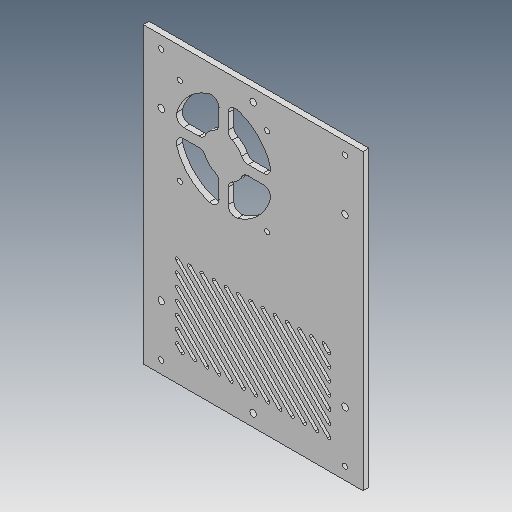
# Autodesk Inventor part: BREEZE-M05
Saved by Autodesk Inventor 2020 (Build 240168000, 168)
## iProperties
Created: 2020-04-12
Part Number: BREEZE-M05
Material: Generic
Description: BOTTOM PANEL
Document SubType Name: Modeling
Designer: John K
Density: 1 g/cm^3
Appearance: Default
Author: John K
Autodesk Inventor part; units mm, degrees
ref_plane "YZ Plane" through (0, 0, 0) normal (1, 0, 0) x (0, 1, 0)
ref_plane "XZ Plane" through (0, 0, 0) normal (0, 1, 0) x (-1, 0, 0)
ref_plane "XY Plane" through (0, 0, 0) normal (0, 0, 1) x (1, 0, 0)
sketch "Face" plane through (0, 0, 0) normal (0, 0, 1) x (1, 0, 0)
  arc A0 (60.9029, -217.5171) -> (63.1656, -215.2543) centre (62.0343, -216.3857) ccw
  arc A1 (29.1656, -161.2543) -> (26.9029, -163.5171) centre (28.0343, -162.3857) ccw
  arc A2 (29.1656, -181.2543) -> (26.9029, -183.5171) centre (28.0343, -182.3857) ccw
  line L0 (29.1656, -191.2543) -> (53.1656, -215.2543)
  arc A3 (50.9029, -217.5171) -> (53.1656, -215.2543) centre (52.0343, -216.3857) ccw
  line L1 (50.9029, -217.5171) -> (26.9029, -193.5171)
  arc A4 (29.1656, -191.2543) -> (26.9029, -193.5171) centre (28.0343, -192.3857) ccw
  line L2 (29.1656, -151.2543) -> (93.1656, -215.2543)
  line L3 (90.9029, -217.5171) -> (26.9029, -153.5171)
  line L4 (60.9029, -217.5171) -> (26.9029, -183.5171)
  line L5 (29.1656, -181.2543) -> (63.1656, -215.2543)
  line L6 (70.9029, -217.5171) -> (26.9029, -173.5171)
  arc A5 (29.1656, -201.2543) -> (26.9029, -203.5171) centre (28.0343, -202.3857) ccw
  line L7 (29.1656, -201.2543) -> (43.1656, -215.2543)
  line L8 (29.1656, -211.2543) -> (33.1656, -215.2543)
  line L9 (30.9029, -217.5171) -> (26.9029, -213.5171)
  line L10 (40.9029, -217.5171) -> (26.9029, -203.5171)
  arc A6 (90.9029, -217.5171) -> (93.1656, -215.2543) centre (92.0343, -216.3857) ccw
  arc A7 (150.9029, -157.5171) -> (153.1656, -155.2543) centre (152.0343, -156.3857) ccw
  line L11 (150.9029, -187.5171) -> (116.9029, -153.5171)
  line L12 (150.9029, -197.5171) -> (106.9029, -153.5171)
  line L13 (109.1656, -151.2543) -> (153.1656, -195.2543)
  line L14 (150.9029, -207.5171) -> (96.9029, -153.5171)
  line L15 (99.1656, -151.2543) -> (153.1656, -205.2543)
  line L16 (89.1656, -151.2543) -> (153.1656, -215.2543)
  line L17 (79.1656, -151.2543) -> (143.1656, -215.2543)
  line L18 (140.9029, -217.5171) -> (76.9029, -153.5171)
  line L19 (130.9029, -217.5171) -> (66.9029, -153.5171)
  line L20 (69.1656, -151.2543) -> (133.1656, -215.2543)
  arc A8 (120.9029, -217.5171) -> (123.1656, -215.2543) centre (122.0343, -216.3857) ccw
  arc A9 (130.9029, -217.5171) -> (133.1656, -215.2543) centre (132.0343, -216.3857) ccw
  arc A10 (140.9029, -217.5171) -> (143.1656, -215.2543) centre (142.0343, -216.3857) ccw
  arc A11 (150.9029, -217.5171) -> (153.1656, -215.2543) centre (152.0343, -216.3857) ccw
  arc A12 (110.9029, -217.5171) -> (113.1656, -215.2543) centre (112.0343, -216.3857) ccw
  arc A13 (150.9029, -187.5171) -> (153.1656, -185.2543) centre (152.0343, -186.3857) ccw
  arc A14 (150.9029, -197.5171) -> (153.1656, -195.2543) centre (152.0343, -196.3857) ccw
  arc A15 (150.9029, -207.5171) -> (153.1656, -205.2543) centre (152.0343, -206.3857) ccw
  circle A16 centre (165.2551, -230.4902) radius 2.1
  line L21 (119.1656, -151.2543) -> (153.1656, -185.2543)
  line L22 (150.9029, -157.5171) -> (146.9029, -153.5171)
  line L23 (149.1656, -151.2543) -> (153.1656, -155.2543)
  line L24 (150.9029, -167.5171) -> (136.9029, -153.5171)
  line L25 (139.1656, -151.2543) -> (153.1656, -165.2543)
  line L26 (129.1656, -151.2543) -> (153.1656, -175.2543)
  arc A17 (150.9029, -167.5171) -> (153.1656, -165.2543) centre (152.0343, -166.3857) ccw
  line L27 (150.9029, -177.5171) -> (126.9029, -153.5171)
  arc A18 (29.1656, -171.2543) -> (26.9029, -173.5171) centre (28.0343, -172.3857) ccw
  circle A19 centre (14.7449, -230.4902) radius 2.1
  arc A20 (30.9029, -217.5171) -> (33.1656, -215.2543) centre (32.0343, -216.3857) ccw
  arc A21 (40.9029, -217.5171) -> (43.1656, -215.2543) centre (42.0343, -216.3857) ccw
  line L28 (180, 0) -> (180, -240.4851)
  line L29 (0, 0) -> (0, -240.4851)
  circle A22 centre (90, -10) radius 2.6
  circle A23 centre (165.25, -188.4851) radius 2.6
  arc A24 (100.9029, -217.5171) -> (103.1656, -215.2543) centre (102.0343, -216.3857) ccw
  circle A25 centre (90, -230.4851) radius 2.6
  arc A26 (80.9029, -217.5171) -> (83.1656, -215.2543) centre (82.0343, -216.3857) ccw
  arc A27 (119.1656, -151.2543) -> (116.9029, -153.5171) centre (118.0343, -152.3857) ccw
  arc A28 (109.1656, -151.2543) -> (106.9029, -153.5171) centre (108.0343, -152.3857) ccw
  arc A29 (70.9029, -217.5171) -> (73.1656, -215.2543) centre (72.0343, -216.3857) ccw
  arc A30 (89.1656, -151.2543) -> (86.9029, -153.5171) centre (88.0343, -152.3857) ccw
  line L30 (0, -240.4851) -> (180, -240.4851)
  arc A31 (79.1656, -151.2543) -> (76.9029, -153.5171) centre (78.0343, -152.3857) ccw
  line L31 (59.1656, -151.2543) -> (123.1656, -215.2543)
  line L32 (120.9029, -217.5171) -> (56.9029, -153.5171)
  arc A32 (69.1656, -151.2543) -> (66.9029, -153.5171) centre (68.0343, -152.3857) ccw
  arc A33 (59.1656, -151.2543) -> (56.9029, -153.5171) centre (58.0343, -152.3857) ccw
  line L33 (49.1656, -151.2543) -> (113.1656, -215.2543)
  line L34 (110.9029, -217.5171) -> (46.9029, -153.5171)
  line L35 (39.1656, -151.2543) -> (103.1656, -215.2543)
  line L36 (100.9029, -217.5171) -> (36.9029, -153.5171)
  line L37 (29.1656, -171.2543) -> (73.1656, -215.2543)
  line L38 (29.1656, -161.2543) -> (83.1656, -215.2543)
  line L39 (80.9029, -217.5171) -> (26.9029, -163.5171)
  arc A34 (49.1656, -151.2543) -> (46.9029, -153.5171) centre (48.0343, -152.3857) ccw
  arc A35 (29.1656, -211.2543) -> (26.9029, -213.5171) centre (28.0343, -212.3857) ccw
  arc A36 (39.1656, -151.2543) -> (36.9029, -153.5171) centre (38.0343, -152.3857) ccw
  arc A37 (29.1656, -151.2543) -> (26.9029, -153.5171) centre (28.0343, -152.3857) ccw
  circle A38 centre (14.75, -188.4851) radius 2.6
  circle A39 centre (14.75, -52) radius 2.6
  arc A40 (139.1656, -151.2543) -> (136.9029, -153.5171) centre (138.0343, -152.3857) ccw
  arc A41 (149.1656, -151.2543) -> (146.9029, -153.5171) centre (148.0343, -152.3857) ccw
  arc A42 (150.9029, -177.5171) -> (153.1656, -175.2543) centre (152.0343, -176.3857) ccw
  arc A43 (99.1656, -151.2543) -> (96.9029, -153.5171) centre (98.0343, -152.3857) ccw
  line L40 (150.9029, -217.5171) -> (86.9029, -153.5171)
  arc A44 (129.1656, -151.2543) -> (126.9029, -153.5171) centre (128.0343, -152.3857) ccw
  circle A45 centre (101.518, -96.0748) radius 2
  circle A46 centre (165.25, -52) radius 2.6
  line L41 (33.2719, -64.3248) -> (45.6124, -64.3248)
  arc A47 (50.9872, -67.6581) -> (45.6124, -64.3248) centre (45.6124, -70.3248) ccw
  arc A48 (33.2719, -64.3248) -> (27.5373, -72.0895) centre (33.2719, -70.3248) ccw
  arc A49 (50.9872, -67.6581) -> (58.6487, -75.2099) centre (65.768, -60.3248) ccw
  arc A50 (62.0599, -80.6227) -> (58.6487, -75.2099) centre (56.0599, -80.6227) ccw
  line L42 (62.0599, -80.6227) -> (62.0599, -92.9094)
  arc A51 (27.5373, -72.0895) -> (54.3467, -98.6596) centre (65.768, -60.3248) ccw
  circle A52 centre (30.018, -96.0748) radius 2
  arc A53 (54.3467, -98.6596) -> (62.0599, -92.9094) centre (56.0599, -92.9094) ccw
  arc A54 (69.4761, -92.9094) -> (77.1893, -98.6596) centre (75.4761, -92.9094) ccw
  line L43 (69.4761, -92.9094) -> (69.4761, -80.6227)
  arc A55 (77.1893, -98.6596) -> (103.9988, -72.0895) centre (65.768, -60.3248) ccw
  arc A56 (72.8873, -75.2099) -> (69.4761, -80.6227) centre (75.4761, -80.6227) ccw
  arc A57 (72.8873, -75.2099) -> (80.5488, -67.6581) centre (65.768, -60.3248) ccw
  arc A58 (103.9988, -72.0895) -> (98.2642, -64.3248) centre (98.2642, -70.3248) ccw
  arc A59 (85.9237, -64.3248) -> (80.5488, -67.6581) centre (85.9237, -70.3248) ccw
  arc A60 (98.2642, -56.3248) -> (103.9988, -48.5601) centre (98.2642, -50.3248) ccw
  arc A61 (77.1893, -21.9901) -> (69.4761, -27.7403) centre (75.4761, -27.7403) ccw
  arc A62 (103.9988, -48.5601) -> (77.1893, -21.9901) centre (65.768, -60.3248) ccw
  line L44 (85.9237, -64.3248) -> (98.2642, -64.3248)
  arc A63 (62.0599, -27.7403) -> (54.3467, -21.9901) centre (56.0599, -27.7403) ccw
  circle A64 centre (14.7449, -9.98) radius 2.1
  circle A65 centre (30.018, -24.5748) radius 2
  circle A66 centre (165.2551, -9.98) radius 2.1
  line L45 (180, 0) -> (0, 0)
  line L46 (98.2642, -56.3248) -> (85.9237, -56.3248)
  arc A67 (80.5488, -52.9915) -> (85.9237, -56.3248) centre (85.9237, -50.3248) ccw
  arc A68 (80.5488, -52.9915) -> (72.8873, -45.4397) centre (65.768, -60.3248) ccw
  arc A69 (69.4761, -40.027) -> (72.8873, -45.4397) centre (75.4761, -40.027) ccw
  line L47 (45.6124, -56.3248) -> (33.2719, -56.3248)
  arc A70 (45.6124, -56.3248) -> (50.9872, -52.9915) centre (45.6124, -50.3248) ccw
  arc A71 (27.5373, -48.5601) -> (33.2719, -56.3248) centre (33.2719, -50.3248) ccw
  arc A72 (58.6487, -45.4397) -> (50.9872, -52.9915) centre (65.768, -60.3248) ccw
  arc A73 (58.6487, -45.4397) -> (62.0599, -40.027) centre (56.0599, -40.027) ccw
  line L48 (62.0599, -27.7403) -> (62.0599, -40.027)
  line L49 (69.4761, -40.027) -> (69.4761, -27.7403)
  circle A74 centre (101.518, -24.5748) radius 2
  arc A75 (54.3467, -21.9901) -> (27.5373, -48.5601) centre (65.768, -60.3248) ccw
  point P0 (82.5578, -141.9576)
  point P1 (4.75, 0)
sketch "Sketch1" plane through (0, 0, 0) normal (0, 0, 1) x (1, 0, 0)
  arc A0 (-29.0971, -97.2745) -> (-26.8344, -95.0118) centre (-27.9657, -96.1432) ccw
  arc A1 (-60.8344, -41.0118) -> (-63.0971, -43.2745) centre (-61.9657, -42.1432) ccw
  arc A2 (-60.8344, -61.0118) -> (-63.0971, -63.2745) centre (-61.9657, -62.1432) ccw
  line L0 (-60.8344, -71.0118) -> (-36.8344, -95.0118)
  arc A3 (-39.0971, -97.2745) -> (-36.8344, -95.0118) centre (-37.9657, -96.1432) ccw
  line L1 (-39.0971, -97.2745) -> (-63.0971, -73.2745)
  arc A4 (-60.8344, -71.0118) -> (-63.0971, -73.2745) centre (-61.9657, -72.1432) ccw
  line L2 (-60.8344, -31.0118) -> (3.1656, -95.0118)
  line L3 (0.9029, -97.2745) -> (-63.0971, -33.2745)
  line L4 (-29.0971, -97.2745) -> (-63.0971, -63.2745)
  line L5 (-60.8344, -61.0118) -> (-26.8344, -95.0118)
  line L6 (-19.0971, -97.2745) -> (-63.0971, -53.2745)
  arc A5 (-60.8344, -81.0118) -> (-63.0971, -83.2745) centre (-61.9657, -82.1432) ccw
  line L7 (-60.8344, -81.0118) -> (-46.8344, -95.0118)
  line L8 (-60.8344, -91.0118) -> (-56.8344, -95.0118)
  line L9 (-59.0971, -97.2745) -> (-63.0971, -93.2745)
  line L10 (-49.0971, -97.2745) -> (-63.0971, -83.2745)
  arc A6 (0.9029, -97.2745) -> (3.1656, -95.0118) centre (2.0343, -96.1432) ccw
  arc A7 (60.9029, -37.2745) -> (63.1656, -35.0118) centre (62.0343, -36.1432) ccw
  line L11 (60.9029, -67.2745) -> (26.9029, -33.2745)
  line L12 (60.9029, -77.2745) -> (16.9029, -33.2745)
  line L13 (19.1656, -31.0118) -> (63.1656, -75.0118)
  line L14 (60.9029, -87.2745) -> (6.9029, -33.2745)
  line L15 (9.1656, -31.0118) -> (63.1656, -85.0118)
  line L16 (-0.8344, -31.0118) -> (63.1656, -95.0118)
  line L17 (-10.8344, -31.0118) -> (53.1656, -95.0118)
  line L18 (50.9029, -97.2745) -> (-13.0971, -33.2745)
  line L19 (40.9029, -97.2745) -> (-23.0971, -33.2745)
  line L20 (-20.8344, -31.0118) -> (43.1656, -95.0118)
  arc A8 (30.9029, -97.2745) -> (33.1656, -95.0118) centre (32.0343, -96.1432) ccw
  arc A9 (40.9029, -97.2745) -> (43.1656, -95.0118) centre (42.0343, -96.1432) ccw
  arc A10 (50.9029, -97.2745) -> (53.1656, -95.0118) centre (52.0343, -96.1432) ccw
  arc A11 (60.9029, -97.2745) -> (63.1656, -95.0118) centre (62.0343, -96.1432) ccw
  arc A12 (20.9029, -97.2745) -> (23.1656, -95.0118) centre (22.0343, -96.1432) ccw
  arc A13 (60.9029, -67.2745) -> (63.1656, -65.0118) centre (62.0343, -66.1432) ccw
  arc A14 (60.9029, -77.2745) -> (63.1656, -75.0118) centre (62.0343, -76.1432) ccw
  arc A15 (60.9029, -87.2745) -> (63.1656, -85.0118) centre (62.0343, -86.1432) ccw
  circle A16 centre (75.2551, -110.2476) radius 2.1
  line L21 (29.1656, -31.0118) -> (63.1656, -65.0118)
  line L22 (60.9029, -37.2745) -> (56.9029, -33.2745)
  line L23 (59.1656, -31.0118) -> (63.1656, -35.0118)
  line L24 (60.9029, -47.2745) -> (46.9029, -33.2745)
  line L25 (49.1656, -31.0118) -> (63.1656, -45.0118)
  line L26 (39.1656, -31.0118) -> (63.1656, -55.0118)
  arc A17 (60.9029, -47.2745) -> (63.1656, -45.0118) centre (62.0343, -46.1432) ccw
  line L27 (60.9029, -57.2745) -> (36.9029, -33.2745)
  arc A18 (-60.8344, -51.0118) -> (-63.0971, -53.2745) centre (-61.9657, -52.1432) ccw
  circle A19 centre (-75.2551, -110.2476) radius 2.1
  arc A20 (-59.0971, -97.2745) -> (-56.8344, -95.0118) centre (-57.9657, -96.1432) ccw
  arc A21 (-49.0971, -97.2745) -> (-46.8344, -95.0118) centre (-47.9657, -96.1432) ccw
  line L28 (90, 120.2425) -> (90, -120.2425)
  line L29 (-90, 120.2425) -> (-90, -120.2425)
  circle A22 centre (0, 110.2425) radius 2.6
  circle A23 centre (75.25, -68.2425) radius 2.6
  arc A24 (10.9029, -97.2745) -> (13.1656, -95.0118) centre (12.0343, -96.1432) ccw
  circle A25 centre (0, -110.2425) radius 2.6
  arc A26 (-9.0971, -97.2745) -> (-6.8344, -95.0118) centre (-7.9657, -96.1432) ccw
  arc A27 (29.1656, -31.0118) -> (26.9029, -33.2745) centre (28.0343, -32.1432) ccw
  arc A28 (19.1656, -31.0118) -> (16.9029, -33.2745) centre (18.0343, -32.1432) ccw
  arc A29 (-19.0971, -97.2745) -> (-16.8344, -95.0118) centre (-17.9657, -96.1432) ccw
  arc A30 (-0.8344, -31.0118) -> (-3.0971, -33.2745) centre (-1.9657, -32.1432) ccw
  line L30 (-90, -120.2425) -> (90, -120.2425)
  arc A31 (-10.8344, -31.0118) -> (-13.0971, -33.2745) centre (-11.9657, -32.1432) ccw
  line L31 (-30.8344, -31.0118) -> (33.1656, -95.0118)
  line L32 (30.9029, -97.2745) -> (-33.0971, -33.2745)
  arc A32 (-20.8344, -31.0118) -> (-23.0971, -33.2745) centre (-21.9657, -32.1432) ccw
  arc A33 (-30.8344, -31.0118) -> (-33.0971, -33.2745) centre (-31.9657, -32.1432) ccw
  line L33 (-40.8344, -31.0118) -> (23.1656, -95.0118)
  line L34 (20.9029, -97.2745) -> (-43.0971, -33.2745)
  line L35 (-50.8344, -31.0118) -> (13.1656, -95.0118)
  line L36 (10.9029, -97.2745) -> (-53.0971, -33.2745)
  line L37 (-60.8344, -51.0118) -> (-16.8344, -95.0118)
  line L38 (-60.8344, -41.0118) -> (-6.8344, -95.0118)
  line L39 (-9.0971, -97.2745) -> (-63.0971, -43.2745)
  arc A34 (-40.8344, -31.0118) -> (-43.0971, -33.2745) centre (-41.9657, -32.1432) ccw
  arc A35 (-60.8344, -91.0118) -> (-63.0971, -93.2745) centre (-61.9657, -92.1432) ccw
  arc A36 (-50.8344, -31.0118) -> (-53.0971, -33.2745) centre (-51.9657, -32.1432) ccw
  arc A37 (-60.8344, -31.0118) -> (-63.0971, -33.2745) centre (-61.9657, -32.1432) ccw
  circle A38 centre (-75.25, -68.2425) radius 2.6
  circle A39 centre (-75.25, 68.2425) radius 2.6
  arc A40 (49.1656, -31.0118) -> (46.9029, -33.2745) centre (48.0343, -32.1432) ccw
  arc A41 (59.1656, -31.0118) -> (56.9029, -33.2745) centre (58.0343, -32.1432) ccw
  arc A42 (60.9029, -57.2745) -> (63.1656, -55.0118) centre (62.0343, -56.1432) ccw
  arc A43 (9.1656, -31.0118) -> (6.9029, -33.2745) centre (8.0343, -32.1432) ccw
  line L40 (60.9029, -97.2745) -> (-3.0971, -33.2745)
  arc A44 (39.1656, -31.0118) -> (36.9029, -33.2745) centre (38.0343, -32.1432) ccw
  circle A45 centre (11.518, 24.1677) radius 2
  circle A46 centre (75.25, 68.2425) radius 2.6
  line L41 (-56.7281, 55.9177) -> (-44.3876, 55.9177)
  arc A47 (-39.0128, 52.5844) -> (-44.3876, 55.9177) centre (-44.3876, 49.9177) ccw
  arc A48 (-56.7281, 55.9177) -> (-62.4627, 48.153) centre (-56.7281, 49.9177) ccw
  arc A49 (-39.0128, 52.5844) -> (-31.3513, 45.0326) centre (-24.232, 59.9177) ccw
  arc A50 (-27.9401, 39.6199) -> (-31.3513, 45.0326) centre (-33.9401, 39.6199) ccw
  line L42 (-27.9401, 39.6199) -> (-27.9401, 27.3332)
  arc A51 (-62.4627, 48.153) -> (-35.6533, 21.583) centre (-24.232, 59.9177) ccw
  circle A52 centre (-59.982, 24.1677) radius 2
  arc A53 (-35.6533, 21.583) -> (-27.9401, 27.3332) centre (-33.9401, 27.3332) ccw
  arc A54 (-20.5239, 27.3332) -> (-12.8107, 21.583) centre (-14.5239, 27.3332) ccw
  line L43 (-20.5239, 27.3332) -> (-20.5239, 39.6199)
  arc A55 (-12.8107, 21.583) -> (13.9988, 48.153) centre (-24.232, 59.9177) ccw
  arc A56 (-17.1127, 45.0326) -> (-20.5239, 39.6199) centre (-14.5239, 39.6199) ccw
  arc A57 (-17.1127, 45.0326) -> (-9.4512, 52.5844) centre (-24.232, 59.9177) ccw
  arc A58 (13.9988, 48.153) -> (8.2642, 55.9177) centre (8.2642, 49.9177) ccw
  arc A59 (-4.0763, 55.9177) -> (-9.4512, 52.5844) centre (-4.0763, 49.9177) ccw
  arc A60 (8.2642, 63.9177) -> (13.9988, 71.6824) centre (8.2642, 69.9177) ccw
  arc A61 (-12.8107, 98.2525) -> (-20.5239, 92.5023) centre (-14.5239, 92.5023) ccw
  arc A62 (13.9988, 71.6824) -> (-12.8107, 98.2525) centre (-24.232, 59.9177) ccw
  line L44 (-4.0763, 55.9177) -> (8.2642, 55.9177)
  arc A63 (-27.9401, 92.5023) -> (-35.6533, 98.2525) centre (-33.9401, 92.5023) ccw
  circle A64 centre (-75.2551, 110.2626) radius 2.1
  circle A65 centre (-59.982, 95.6677) radius 2
  circle A66 centre (75.2551, 110.2626) radius 2.1
  line L45 (90, 120.2425) -> (-90, 120.2425)
  line L46 (8.2642, 63.9177) -> (-4.0763, 63.9177)
  arc A67 (-9.4512, 67.2511) -> (-4.0763, 63.9177) centre (-4.0763, 69.9177) ccw
  arc A68 (-9.4512, 67.2511) -> (-17.1127, 74.8028) centre (-24.232, 59.9177) ccw
  arc A69 (-20.5239, 80.2156) -> (-17.1127, 74.8028) centre (-14.5239, 80.2156) ccw
  line L47 (-44.3876, 63.9177) -> (-56.7281, 63.9177)
  arc A70 (-44.3876, 63.9177) -> (-39.0128, 67.2511) centre (-44.3876, 69.9177) ccw
  arc A71 (-62.4627, 71.6824) -> (-56.7281, 63.9177) centre (-56.7281, 69.9177) ccw
  arc A72 (-31.3513, 74.8028) -> (-39.0128, 67.2511) centre (-24.232, 59.9177) ccw
  arc A73 (-31.3513, 74.8028) -> (-27.9401, 80.2156) centre (-33.9401, 80.2156) ccw
  line L48 (-27.9401, 92.5023) -> (-27.9401, 80.2156)
  line L49 (-20.5239, 80.2156) -> (-20.5239, 92.5023)
  circle A74 centre (11.518, 95.6677) radius 2
  arc A75 (-35.6533, 98.2525) -> (-62.4627, 71.6824) centre (-24.232, 59.9177) ccw
  point P0 (0, 0)
  point P1 (-90, 0)
  point P2 (0, 120.2425)
  constraints: 1 horizontal alignment, 1 vertical alignment, 2 other
extrude "Extrusion1" add sketch "Sketch1" along normal mid plane 4.75
body "Solid1"
